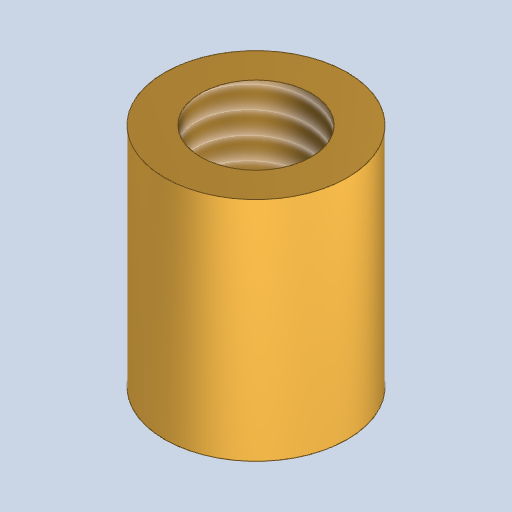
# Autodesk Inventor part: BRM2-4.1
Saved by Autodesk Inventor 2022.3 (Build 263350000, 350)
## iProperties
Part Number: BRM2-4.1
Material: 真鍮、ソフト イエロー
Document SubType Name: Modeling
Designer: Masato Kubotera
Density: 8.47 g/cm^3
Appearance: 真鍮 - サテン
Catalog Web Link: https://jp.misumi-ec.com/vona2/detail/221005351346/?HissuCode=BRM2-4.1
Description: ReadyMade
Author: Masato Kubotera
Autodesk Inventor part; units mm, degrees
ref_plane "YZ Plane" through (0, 0, 0) normal (1, 0, 0) x (0, 1, 0)
ref_plane "XZ Plane" through (0, 0, 0) normal (0, 1, 0) x (-1, 0, 0)
ref_plane "XY Plane" through (0, 0, 0) normal (0, 0, 1) x (1, 0, 0)
sketch "スケッチ1" plane through (0, 0, 0) normal (0, 1, 0) x (-1, 0, 0)
  line L0 (-1, 0) -> (-1.65, 0)
  line L1 (-1.65, 0) -> (-1.65, 4.1)
  line L2 (-1.65, 4.1) -> (-1, 4.1)
  line L3 (-1, 4.1) -> (-1, 0)
  line L4 (0, 0) -> (0, 4.1) construction
  dimension "d0" = 3.3
  dimension "d1" = 2
  dimension "d2" = 4.1
  constraints: 10 end point, 2 parallel, 2 point on line, 1 horizontal, 1 perpendicular, 1 vertical
  measures "d0" diameter of L1 L4
  measures "d1" diameter of L3 L4
  measures "d2" distance of L0.end L1.end
revolve "回転1" add sketch "スケッチ1" angle 360 about axis through (0, 0, 0) along (0, 0, 1)
thread "ねじ1" size "M2x0.4" class "6H" standard "ANSI Metric M Profile" full length
